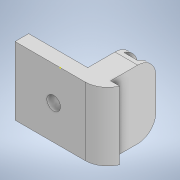
# Autodesk Inventor part: Peça2
Saved by Autodesk Inventor 2022 (Build 260153000, 153)
## iProperties
Created: 2023-10-22
Part Number: Peça2
Material: Genérico
Document SubType Name: Modeling
Designer: Daniel
Density: 1 g/cm^3
Appearance: Padrão
Author: Daniel
Autodesk Inventor part; units mm, degrees
ref_plane "YZ Plane" through (0, 0, 0) normal (1, 0, 0) x (0, 1, 0)
ref_plane "XZ Plane" through (0, 0, 0) normal (0, 1, 0) x (-1, 0, 0)
ref_plane "XY Plane" through (0, 0, 0) normal (0, 0, 1) x (1, 0, 0)
sketch "Esboço1" plane through (0, 0, 0) normal (0, 0, 1) x (1, 0, 0)
  line L0 (-10, 7.5) -> (10, 7.5)
  line L1 (10, 7.5) -> (10, -7.5)
  line L2 (10, -7.5) -> (-10, -7.5)
  line L3 (-10, -7.5) -> (-10, 7.5)
  line L4 (-10, 7.5) -> (10, -7.5) construction
  line L5 (10, 7.5) -> (-10, -7.5) construction
  circle A0 centre (-1.5, 0) radius 1.5
  point P0 (0, 0)
  dimension "d0" = 20
  dimension "d1" = 15
  dimension "d13" = 3
  dimension "d14" = 1.5
  dimension "d15" = 7.5
  constraints: 12 end point, 2 midpoint, 2 parallel, 1 centre point, 1 horizontal, 1 perpendicular
  measures "d0" distance of L0.start L0.end
  measures "d1" distance of L2.end L0.start
  measures "d13" diameter of A0
  measures "d14" distance of point (0, 0) A0.centre
  measures "d15" distance from line of L2 A0.centre
extrude "Extrusão1" add sketch "Esboço1" against normal blind 3
sketch "Esboço2" plane through (0, 0, -3) normal (0, 0, -1) x (-1, 0, 0)
  line L0 (10, 7.5) -> (-10, 7.5) projected
  line L1 (-4, 7.5) -> (-4, -7.5247)
  line L2 (-7, 7.5) -> (-7, -7.5)
  line L3 (-10, -7.5) -> (10, -7.5) projected
  line L4 (-3, 7.5) -> (-3, -7.5247)
  line L5 (-8, 7.5) -> (-8, -7.5)
  point P0 (0, 0)
  point P1 (0, 0)
  point P2 (-3, -7.5)
  point P3 (-4, -7.5)
  dimension "d6" = 3
  dimension "d7" = 1
  dimension "d8" = 1
  dimension "d16" = 7
  constraints: 8 end point, 3 point on line, 2 parallel, 2 vertical
  measures "d6" distance between parallel lines of L2 L1
  measures "d7" distance between parallel lines of L1 L4
  measures "d8" distance between parallel lines of L2 L5
  measures "d16" horizontal distance of L2.start point (0, 0)
extrude "Extrusão2" add sketch "Esboço2" along normal blind 10 contours L4 L3 L1 L0 | L2 L3 L5 L0
sketch "Esboço3" plane through (-10, 7.5, 0) normal (0, 1, 0) x (1, 0, 0)
  point P0 (10, 0)
fillet "Arredondamento1" radius 5 1 edges at (10, 0, 0)
sketch "Esboço4" plane through (0, 0, -3) normal (0, 0, -1) x (-1, 0, 0)
  line L0 (-7, 7.5) -> (-7, -7.5) projected
  line L1 (-7, -7.5) -> (-4, -7.5) projected
  line L2 (-4, -7.5) -> (-4, 7.5) projected
  line L3 (-4, 7.5) -> (-7, 7.5) projected
  point P0 (0, 0)
extrude "Extrusão3" add sketch "Esboço4" along normal blind 7
fillet "Arredondamento3" radius 4 4 edges at (3.5, 7.5, -13) (7.5, 7.5, -13) (3.5, -7.5, -13) (7.5, -7.5, -13)
